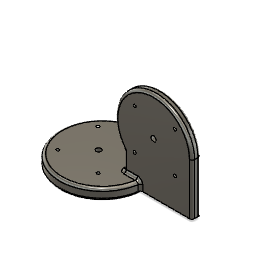
full_robot v3 (Autodesk Fusion 360 archive; units mm, degrees)
design "Cintura"
Autodesk Fusion 360 part; units mm, degrees
sketch "Sketch1" plane through (0, 0, 0) normal (0, 1, 0) x (1, 0, 0)
  circle A0 centre (0, 0) radius 50
  dimension "d1" = 100
  constraint coincident A0.centre origin
  measures "d1" diameter of A0
extrude "Extrude1" add sketch "Sketch1" along normal blind 10
sketch "Sketch2" plane through (0, 0, 0) normal (0, 1, 0) x (1, 0, 0)
  circle A0 centre (0, 0) radius 47.5
  dimension "d4" = 95
  constraint coincident A0.centre origin
  measures "d4" diameter of A0
extrude "Extrude2" add sketch "Sketch2" against normal blind 3
sketch "Sketch3" plane through (0, 0, 0) normal (0, 0, 1) x (1, 0, 0)
  line L0 (30, 0) -> (110, 0)
  line L1 (110, 0) -> (110, 50)
  line L2 (110, 50) -> (110, 60)
  arc A0 (110, 60) -> (30, 31.7157) centre (65, 60) ccw
  line L3 (30, 31.7157) -> (30, 0)
  dimension "d7" = 80
  dimension "d8" = 50
  dimension "d9" = 45
  dimension "d10" = 30
  dimension "d11" = 60
  constraint horizontal L0
  constraint perpendicular L0 L1
  constraint parallel L1 L2
  constraint tangent L2 A0
  constraint perpendicular L0 L3
  measures "d7" distance of L0.start L0.end
  measures "d8" distance of L0.end L1.end
  measures "d9" radius of A0
  measures "d10" distance of origin L0.start
  measures "d11" vertical distance of origin A0.centre
extrude "Extrude3" add sketch "Sketch3" along normal mid plane 10
sketch "Sketch4" plane through (0, 0, -5) normal (0, 0, -1) x (-1, 0, 0)
  line L0 (-49.7494, 10) -> (-30, 10)
  line L1 (-30, 10) -> (-30, 31.7157)
  arc A0 (-30, 31.7157) -> (-110, 60) centre (-65, 60) ccw
  line L2 (-110, 60) -> (-110, 0)
  line L3 (-110, 0) -> (-49.7494, 0)
  line L4 (-49.7494, 0) -> (-49.7494, 10)
  line L5 (-90, 82.244) -> (-42.756, 82.244)
  line L6 (-42.756, 82.244) -> (-42.756, 35)
  line L7 (-42.756, 35) -> (-90, 35)
  line L8 (-90, 35) -> (-90, 82.244)
  dimension "d14" = 47.244
  dimension "d15" = 47.244
  dimension "d16" = 25
  dimension "d17" = 25
  constraint horizontal L5
  constraint vertical L6
  constraint horizontal L7
  constraint vertical L8
  measures "d14" distance of L5.start L5.end
  measures "d15" distance of L5.start L7.end
  measures "d16" horizontal distance of A0.centre L7.end
  measures "d17" vertical distance of A0.centre L7.end
hole "Hole1" at (90, 82.244, -5) at (42.756, 82.244, -5) at (42.756, 35, -5) at (90, 35, -5) direction (0, 0, 1) diameter 3.332 end through all
hole "Hole2" at (65, 60, -5) direction (0, 0, 1) diameter 6 depth 10 tip angle 118
sketch "Sketch5" plane through (0, 10, 0) normal (0, 1, 0) x (-1, 0, 0)
  line L0 (-49.7494, 5) -> (-30, 5)
  line L1 (-30, 5) -> (-30, -5)
  line L2 (-30, -5) -> (-49.7494, -5)
  arc A0 (-49.7494, -5) -> (-49.7494, 5) centre (0, 0) ccw
  line L3 (30, -25) -> (-17.244, -25)
  line L4 (-17.244, -25) -> (-17.244, 22.244)
  line L5 (-17.244, 22.244) -> (30, 22.244)
  line L6 (30, 22.244) -> (30, -25)
  dimension "d24" = 47.244
  dimension "d25" = 47.244
  dimension "d26" = 30
  dimension "d27" = 25
  constraint horizontal L3
  constraint vertical L4
  constraint horizontal L5
  constraint vertical L6
  measures "d24" distance of L3.start L3.end
  measures "d25" distance of L3.start L5.end
  measures "d26" horizontal distance of A0.centre L3.start
  measures "d27" vertical distance of A0.centre L3.end
hole "Hole3" at (-30, 10, -25) at (17.244, 10, -25) at (17.244, 10, 22.244) at (-30, 10, 22.244) direction (0, -1, 0) diameter 3.332 depth 8 tip angle 118
thread "Thread1" "ISO Metric profile 4.0 M4x0.7 6H" major diameter 4.1095 minor diameter 3.332 pitch 0.7 angle 60 resizes the face on face at (16.1731, 7.3333, -26.2762) on face at (-31.0709, 7.3333, 20.9678) on face at (16.1731, 7.3333, 20.9678) on face at (-31.0709, 7.3333, -26.2762)
hole "Hole4" at (-5.9773, 10, -1.5751) direction (0, -1, 0) diameter 6 end through all
fillet "Fillet1" radius 3 1 edges at (-50, 10, 0)
fillet "Fillet2" radius 3 4 edges at (50, 102.4264, -5) (110, 30, -5) (110, 30, 5) (50, 102.4264, 5)
fillet "Fillet3" radius 3 2 edges at (30, 23.3918, -5) (30, 23.3918, 5)
fillet "Fillet4" radius 3 9 edges at (49.7494, 3.5, 5) (48.8635, 9.124, 5) (39.8666, 10, 5) (30.8787, 10, 4.1213) (30, 10, 0) (30.8787, 10, -4.1213) (39.8666, 10, -5) (48.8635, 9.124, -5) (49.7494, 3.5, -5)

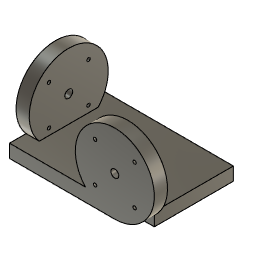
design "4-conexao_braco_punho"
Autodesk Fusion 360 part; units mm, degrees
sketch "Sketch1" plane through (0, 0, 0) normal (0, 0, 1) x (1, 0, 0)
  line L0 (-25, 50) -> (75, 50)
  line L1 (75, 50) -> (75, -20)
  line L2 (75, -20) -> (-25, -20)
  line L3 (-25, -20) -> (-25, 50)
  dimension "d1" = 100
  dimension "d2" = 70
  constraint horizontal L0
  constraint vertical L1
  constraint horizontal L2
  constraint vertical L3
  measures "d1" distance of L0.start L0.end
  measures "d2" distance of L0.start L2.end
extrude "Extrude1" add sketch "Sketch1" along normal blind 10
sketch "Sketch2" plane through (0, 0, 0) normal (1, 0, 0) x (0, 1, 0)
  line L0 (-20, 50) -> (-20, -25) construction
  line L1 (50, 50) -> (50, -25) construction
  line L2 (-25, 0) -> (55, 0) construction
  line L3 (15, 50) -> (15, -25) construction
  line L4 (-25, 30) -> (55, 30) construction
  circle A0 centre (15, 30) radius 3
  circle A1 centre (15, 30) radius 30
  circle A2 centre (0, 15) radius 1.265
  circle A3 centre (15, 30) radius 3
  circle A4 centre (0, 45) radius 1.265
  circle A5 centre (30, 45) radius 1.265
  circle A6 centre (15, 30) radius 3
  circle A7 centre (30, 15) radius 1.265
  circle A8 centre (15, 30) radius 3
  line L5 (59.9207, 15) -> (-20, 15) construction
  line L6 (30, 60) -> (30, -2) construction
  line L7 (0, 60) -> (0, -2) construction
  point P0 (0, 45)
  dimension "d5" = 35
  dimension "d6" = 30
  dimension "d7" = 6
  dimension "d8" = 60
  dimension "d9" = 2.53
  dimension "d10" = 2.53
  dimension "d18" = 15
  dimension "d19" = 15
  constraint vertical L0
  constraint vertical L1
  constraint perpendicular L1 L2
  constraint perpendicular L2 L3
  constraint perpendicular L1 L4
  constraint concentric A0 A1
  constraint symmetric L4 A0 A3
  constraint symmetric L4 A2.centre P0
  constraint coincident P0 A4.centre
  constraint symmetric L3 A3 A6
  constraint symmetric L3 A4 A5
  constraint symmetric L3 A2 A7
  constraint symmetric L3 A3 A8
  constraint coincident L0 L5.end
  constraint perpendicular L0 L5
  constraint perpendicular L2 L6
  constraint perpendicular L2 L7
  measures "d5" distance of L0 L3
  measures "d6" distance of L2 L4
  measures "d7" diameter of A0
  measures "d8" diameter of A1
  measures "d9" diameter of A2
  measures "d10" diameter of A4
  measures "d18" distance of L4 L5
  measures "d19" distance of L3 L7
extrude "Extrude2" add sketch "Sketch2" along normal blind 10 from surface at -25
sketch "Sketch3" plane through (0, 0, 0) normal (0, 1, 0) x (1, 0, 0)
  line L0 (-30, 0) -> (80, 0) construction
  line L1 (25, -65) -> (25, 5) construction
  line L2 (-30, -30) -> (80, -30) construction
  line L3 (-25, -65) -> (-25, 5) construction
  circle A0 centre (55, -30) radius 30
  circle A1 centre (55, -30) radius 3
  line L4 (-35, -15) -> (111.1834, -15) construction
  line L5 (55, -65) -> (55, 5) construction
  line L6 (70, -70) -> (70, 15) construction
  circle A2 centre (70, -15) radius 1.265
  circle A3 centre (55, -30) radius 3
  circle A4 centre (70, -45) radius 1.265
  circle A5 centre (55, -30) radius 3
  circle A6 centre (40, -15) radius 1.265
  circle A7 centre (55, -30) radius 3
  circle A8 centre (40, -45) radius 1.265
  point P0 (70, -45)
  point P1 (40, -15)
  point P2 (40, -45)
  dimension "d14" = 50
  dimension "d15" = 30
  dimension "d16" = 60
  dimension "d17" = 6
  dimension "d20" = 15
  dimension "d21" = 15
  dimension "d22" = 2.53
  dimension "d23" = 2.53
  dimension "d24" = 2.53
  dimension "d25" = 2.53
  constraint horizontal L0
  constraint perpendicular L0 L1
  constraint horizontal L2
  constraint perpendicular L0 L3
  constraint coincident L2 A0.centre
  constraint concentric A0 A1
  constraint horizontal L4
  constraint perpendicular L0 L5
  constraint vertical L6
  constraint coincident L6 A2.centre
  constraint coincident L4 A2.centre
  constraint symmetric L2 A1 A3
  constraint symmetric L2 A2.centre P0
  constraint coincident P0 A4.centre
  constraint symmetric L5 A2.centre P1
  constraint symmetric L5 A3 A5
  constraint coincident P1 A6.centre
  constraint symmetric L2 A5 A7
  constraint symmetric L2 P1 P2
  constraint coincident P2 A8.centre
  measures "d14" distance of L1 L3
  measures "d15" distance of L0 L2
  measures "d16" diameter of A0
  measures "d17" diameter of A1
  measures "d20" distance of L2 L4
  measures "d21" distance of L5 L6
  measures "d22" diameter of A2
  measures "d23" diameter of A4
  measures "d24" diameter of A6
  measures "d25" diameter of A8
extrude "Extrude3" add sketch "Sketch3" along normal blind 10 from surface at -20
ref_plane "WorkPlane1" through (0, -30, 0) normal (0, 1, 0) x (0, 0, 1)
sketch "Sketch4" plane through (0, -30, 0) normal (0, 1, 0) x (1, 0, 0)
  line L0 (85, 0) -> (-35, 0) construction
  line L1 (-35, -7.64) -> (92.4851, -7.64) construction
  circle A0 centre (55, -30) radius 30 construction
  line L2 (55, -30) -> (55, 12) construction
  line L3 (75.0008, -7.64) -> (75.0008, 0)
  line L4 (55, 0) -> (75.0008, 0)
  circle A1 centre (55, -30) radius 30
  dimension "d30" = 60
  constraint horizontal L0
  constraint horizontal L1
  constraint perpendicular L1 L2
  constraint coincident A0 L3.start
  constraint coincident L1 L3.start
  constraint perpendicular L1 L3
  constraint coincident A0 L4.start
  constraint coincident L0 L4.start
  constraint perpendicular L2 L4
  constraint concentric A0 A1
  constraint coincident L3.start A1
  measures "d30" diameter of A0
extrude "Extrude4" cut sketch "Sketch4" along normal blind 10 from surface at 10 contours L3 L4 A1

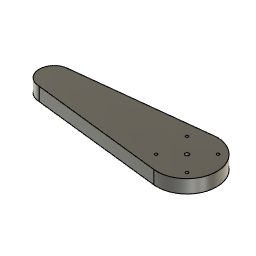
design "3-braco-2"
Autodesk Fusion 360 part; units mm, degrees
sketch "Sketch1" plane through (0, 0, 0) normal (0, 0, 1) x (1, 0, 0)
  circle A0 centre (-74.4665, 27.0941) radius 22.5
  line L0 (-74.4665, 27.0941) -> (-74.4665, 117.7427) construction
  line L1 (125.5335, 27.0941) -> (125.5335, 120) construction
  line L2 (-74.4665, 27.0941) -> (124.443, 27.0941) construction
  line L3 (25.5335, 130) -> (25.5335, -85.9983) construction
  circle A1 centre (125.5335, 27.0941) radius 45
  line L4 (-74.4665, 49.5941) -> (125.5335, 72.0941)
  line L5 (-74.3843, 4.5942) -> (120.4363, -17.6163)
  circle A2 centre (125.5335, 27.3791) radius 3
  circle A3 centre (102.199, 50.7137) radius 1.665
  circle A4 centre (102.199, 4.0446) radius 1.665
  circle A5 centre (149.443, 3.4697) radius 1.665
  circle A6 centre (148.868, 50.7137) radius 1.665
  line L6 (102.199, 50.7137) -> (149.443, 50.7137)
  line L7 (149.443, 50.7137) -> (149.443, 3.4697)
  line L8 (149.443, 3.4697) -> (102.199, 3.4697)
  line L9 (102.199, 3.4697) -> (102.199, 50.7137)
  point P0 (125.5335, 27.3791)
  point P1 (125.5335, 27.3791)
  dimension "d1" = 45
  dimension "d3" = 200
  dimension "d4" = 100
  dimension "d6" = 33
  dimension "d9" = 6
  dimension "d10" = 3.33
  dimension "d11" = 3.33
  dimension "d12" = 3.33
  dimension "d13" = 3.33
  dimension "d14" = 90
  dimension "d15" = 47.244
  dimension "d16" = 47.244
  constraint coincident A0.centre L0.start
  constraint vertical L0
  constraint vertical L1
  constraint perpendicular L0 L2
  constraint vertical L3
  constraint coincident P1 P0
  constraint coincident L1.start A1.centre
  constraint coincident A0 L4.start
  constraint coincident L0 L4.start
  constraint coincident A1 L4.end
  constraint coincident L1 L4.end
  constraint coincident A0 L5.start
  constraint coincident A1 L5.end
  constraint tangent A1 L5
  constraint horizontal L6
  constraint vertical L7
  constraint horizontal L8
  constraint vertical L9
  constraint coincident A5.centre L7.end
  constraint coincident A3.centre L6.start
  measures "d1" diameter of A0
  measures "d3" distance of A0.centre L1.start
  measures "d4" distance of L0 L3
  measures "d6" distance of P1 A6.centre
  measures "d9" diameter of A2
  measures "d10" diameter of A3
  measures "d11" diameter of A4
  measures "d12" diameter of A5
  measures "d13" diameter of A6
  measures "d14" diameter of A1
  measures "d15" distance of A3.centre L6.end
  measures "d16" distance of L6.end A5.centre
extrude "Extrude1" add sketch "Sketch1" against normal blind 20 contours A0 | A0 A1 L4 L5 | A1 L4 | A2 | A3 L6 L9 | A3 A4 A5 A6 L6 L7 L8 L9 | A3 L6 L9 | A6 L6 L7 | A6 L6 L7 | A4 L8 L9 | A4 L8 L9 | A5 L7 L8 | A5 L7 L8 picked at (94.9797, 27.5619)
hole "Hole1" at (102.199, 50.7137, 0) at (102.199, 4.0446, 0) at (149.443, 3.4697, 0) at (148.868, 50.7137, 0) direction (0, 0, -1) diameter 4 depth 10 tip angle 118
extrude "Extrude2" cut sketch "Sketch1" against normal blind 6 contours A2

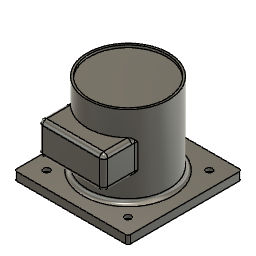
design "Base"
Autodesk Fusion 360 part; units mm, degrees
sketch "Sketch1" plane through (0, 0, 0) normal (0, 1, 0) x (1, 0, 0)
  line L0 (70, -70) -> (-70, -70)
  line L1 (-70, -70) -> (-70, 70)
  line L2 (-70, 70) -> (70, 70)
  line L3 (70, 70) -> (70, -70)
  line L4 (70, -70) -> (-70, 70) construction
  line L5 (-70, -70) -> (70, 70) construction
  dimension "d1" = 140
  dimension "d2" = 140
  constraint horizontal L0
  constraint perpendicular L0 L1
  constraint parallel L0 L2
  constraint parallel L1 L3
  constraint coincident L4 origin
  constraint coincident L5 origin
  measures "d1" distance of L1.end L2.end
  measures "d2" distance of L0.end L1.end
extrude "Extrude1" add sketch "Sketch1" along normal blind 10
sketch "Sketch2" plane through (0, 10, 0) normal (0, 1, 0) x (-1, 0, 0)
  line L0 (-70, -70) -> (70, -70)
  line L1 (70, -70) -> (70, 70)
  line L2 (70, 70) -> (-70, 70)
  line L3 (-70, 70) -> (-70, -70)
  circle A0 centre (0, 0) radius 50
  dimension "d5" = 100
  constraint coincident A0.centre origin
  measures "d5" diameter of A0
extrude "Extrude2" add sketch "Sketch2" along normal blind 100 contours A0
sketch "Sketch3" plane through (0, 0, 0) normal (0, 0, 1) x (1, 0, 0)
  line L0 (-40, 80) -> (40, 80)
  line L1 (40, 80) -> (40, 40)
  line L2 (40, 40) -> (-40, 40)
  line L3 (-40, 40) -> (-40, 80)
  dimension "d8" = 80
  dimension "d9" = 40
  dimension "d10" = 40
  dimension "d11" = 40
  constraint horizontal L0
  constraint vertical L1
  constraint horizontal L2
  constraint vertical L3
  measures "d8" distance of L0.start L0.end
  measures "d9" distance of L0.start L2.end
  measures "d10" horizontal distance of origin L2.end
  measures "d11" distance of origin L2
extrude "Extrude3" add sketch "Sketch3" along normal blind 70
sketch "Sketch4" plane through (0, 110, 0) normal (0, 1, 0) x (-1, 0, 0)
  circle A0 centre (0, 0) radius 50
  circle A1 centre (0, 0) radius 47.5
  dimension "d14" = 95
  constraint coincident A0.centre A1.centre
  measures "d14" diameter of A1
extrude "Extrude4" cut sketch "Sketch4" against normal blind 3 contours A1
sketch "Sketch5" plane through (0, 10, 0) normal (0, 1, 0) x (-1, 0, 0)
  circle A0 centre (0, 0) radius 50
  line L0 (-70, -70) -> (70, -70)
  line L1 (70, -70) -> (70, 70)
  line L2 (70, 70) -> (-70, 70)
  line L3 (-70, 70) -> (-70, -70)
  point P0 (50, -50)
  point P1 (-50, -50)
  point P2 (-50, 50)
  point P3 (50, 50)
  dimension "d17" = 20
  dimension "d18" = 20
  dimension "d19" = 20
  dimension "d20" = 20
  dimension "d21" = 20
  dimension "d22" = 20
  dimension "d23" = 20
  dimension "d24" = 20
  measures "d17" horizontal distance of L0.end P0
  measures "d18" vertical distance of L0.end P0
  measures "d19" horizontal distance of L0.start P1
  measures "d20" vertical distance of L0.start P1
  measures "d21" horizontal distance of L2.end P2
  measures "d22" vertical distance of L2.end P2
  measures "d23" horizontal distance of L1.end P3
  measures "d24" vertical distance of L1.end P3
hole "Hole1" at (50, 10, -50) at (-50, 10, -50) at (-50, 10, 50) at (50, 10, 50) direction (0, -1, 0) diameter 4.5 depth 40 tip angle 118 counterbore diameter 8 counterbore depth 4
fillet "Fillet1" radius 3 4 edges at (70, 5, 70) (-70, 5, 70) (70, 5, -70) (-70, 5, -70)
fillet "Fillet2" radius 5 4 edges at (40, 60, 30) (40, 60, 70) (-40, 60, 70) (-40, 60, 30)
fillet "Fillet3" radius 5 14 edges at (40.2327, 80, 30.1152) (40, 80, 48.3114) (38.5355, 80, 68.5355) (0, 80, 70) (-38.5355, 80, 68.5355) (-40, 80, 48.3114) (-40.2327, 80, 30.1152) (-40.2327, 40, 30.1152) (-40, 40, 48.3114) (-38.5355, 40, 68.5355) (0, 40, 70) (38.5355, 40, 68.5355) (40, 40, 48.3114) (40.2327, 40, 30.1152)
fillet "Fillet4" radius 5 1 edges at (46.6164, 10, 18.0808)
